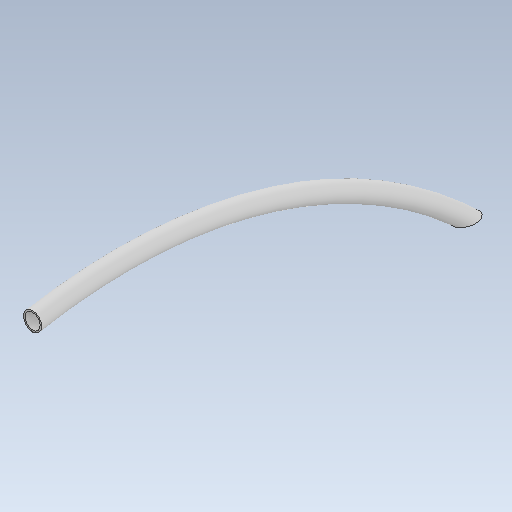
# Autodesk Inventor part: large_hoop
Saved by Autodesk Inventor 2021 (Build 250183000, 183)
## iProperties
Created: 2021-05-05
Part Number: large_hoop
Material: Generic
Document SubType Name: Modeling
Density: 1 g/cm^3
Appearance: Default
Autodesk Inventor part; units mm, degrees
ref_plane "YZ Plane" through (0, 0, 0) normal (1, 0, 0) x (0, 1, 0)
ref_plane "XZ Plane" through (0, 0, 0) normal (0, 1, 0) x (-1, 0, 0)
ref_plane "XY Plane" through (0, 0, 0) normal (0, 0, 1) x (1, 0, 0)
sketch "Sketch1" plane through (0, 0, 0) normal (1, 0, 0) x (0, 1, 0)
  circle A0 centre (0, 0) radius 1650
  dimension "d0" = 3300
  constraints: 1 centre point, 1 coincident
  measures "d0" diameter of A0
sketch "Sketch2" plane through (0, 0, 0) normal (0, 0, 1) x (1, 0, 0)
  circle A0 centre (0, 1650) radius 30
  point P0 (0, 0)
  dimension "d1" = 1650
  dimension "d2" = 0
  dimension "d3" = 60
  constraints: 1 centre point
  measures "d1" distance of A0.centre point (0, 0)
  measures "d2" horizontal distance of A0.centre point (0, 0)
  measures "d3" diameter of A0
sweep "Sweep1" add profiles "Sketch2" path "Sketch1"
sketch "Sketch3" plane through (0, 0, 0) normal (0, 0, 1) x (1, 0, 0)
  circle A0 centre (0, 1650) radius 25
  point P0 (0, 0)
  dimension "d6" = 50
  dimension "d7" = 0
  dimension "d8" = 1650
  constraints: 1 centre point
  measures "d6" diameter of A0
  measures "d7" horizontal distance of A0.centre point (0, 0)
  measures "d8" distance of point (0, 0) A0.centre
sweep "Sweep2" cut profiles "Sketch3" path "Sketch1"
sketch "Sketch4" plane through (0, 0, 0) normal (1, 0, 0) x (0, 1, 0)
  line L0 (1200, 1730) -> (1200, -1730)
  line L1 (1200, 300) -> (2930, 300)
  line L2 (2930, 300) -> (2930, 1730)
  line L3 (1200, 1730) -> (1330.0646, 1730)
  line L4 (1330.0646, 1730) -> (2930, 1730)
  line L5 (1200, 1730) -> (-1730, 1730)
  line L6 (-1730, 1730) -> (-1730, -1730)
  line L7 (-1730, -1730) -> (1200, -1730)
  point P0 (0, 0)
  dimension "d12" = 3460
  dimension "d13" = 1730
  dimension "d14" = 1200
  dimension "d15" = 1730
  dimension "d16" = 1730
  dimension "d17" = 300
  constraints: 17 end point, 2 horizontal, 2 perpendicular, 2 point on line, 2 vertical
  measures "d12" distance of L0.start L0.end
  measures "d13" vertical distance of point (0, 0) L0.start
  measures "d14" distance from line of point (0, 0) L0
  measures "d15" distance from line of point (0, 0) L6
  measures "d16" distance of L1.start L1.end
  measures "d17" distance from line of point (0, 0) L1
extrude "Extrusion1" cut sketch "Sketch4" along normal mid plane 80
sketch "Sketch5" plane through (0, 0, 0) normal (1, 0, 0) x (0, 1, 0)
  line L0 (1591.9799, 300) -> (1593.8318, 290.173)
  circle A0 centre (0, 0) radius 1620
  line L1 (1652.9973, 300) -> (1591.9799, 300) projected
  line L2 (1591.9799, 300) -> (1590.9972, 299.8148)
  line L3 (1590.9972, 299.8148) -> (1592.849, 289.9878)
  arc A1 (1200, -1088.3014) -> (1591.9799, 300) centre (0, 0) ccw projected
  line L4 (1593.8318, 290.173) -> (1592.849, 289.9878)
  point P0 (1593.8014, 290.1672)
  point P1 (500, 900)
  dimension "d20" = 10
  dimension "d21" = 10
  dimension "d22" = 1
  constraints: 8 end point, 2 perpendicular, 1 coincident, 1 point on line, 6 other
  measures "d20" distance of L0.start L0.end
  measures "d21" distance of L2.end L3.end
  measures "d22" distance of L2.start L2.end
extrude "Extrusion2" add sketch "Sketch5" against normal mid plane 10 contours A0 L4 L3 L2 picked at (1592.3491, 294.4162)
equation "\"d0\" = hoop_radius_large"
equation "\"d1\" = 0.5 * d0"
equation "\"d3\" = hoop_width_medium"
equation "\"d6\" = hoop_width_medium - hoop_thickness_medium"
equation "\"d8\" = 0.5 * d0"
equation "\"d12\" = 2 * hoop_width_large + d0"
equation "\"d13\" = 0.5 * d12"
equation "\"d14\" = 0.5 * hoop_radius_large - hoop_height_large"
equation "\"d15\" = 0.5 * d12"
equation "\"d16\" = d13"
equation "\"d17\" = hoop_length_large"
equation "\"d18\" = hoop_width_large"
equation "\"d21\" = d20"
equation "\"rack_tooth_thickness\" = 5"
equation "\"rack_tooth_addendum\" = 5"
equation "\"rack_tooth_dedendum\" = 5"
equation "\"hoop_radius_large\" = 3300"
equation "\"hoop_width_large\" = 80"
equation "\"hoop_width_medium\" = 60"
equation "\"hoop_thickness_medium\" = 10"
equation "\"hoop_length_large\" = 300"
equation "\"hoop_height_large\" = 450"
body "Solid1"
